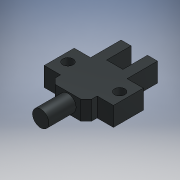
# Autodesk Inventor part: RX670-NW
Saved by Autodesk Inventor 2017 (Build 210142000, 142)
## iProperties
Part Number: RX670-NW
Material: SS41
Document SubType Name: Modeling
Designer: G
Density: 7.85 g/cm^3
Appearance: 鐵灰色
Author: G
Autodesk Inventor part; units mm, degrees
ref_plane "YZ Plane" through (0, 0, 0) normal (1, 0, 0) x (0, 1, 0)
ref_plane "XZ Plane" through (0, 0, 0) normal (0, 1, 0) x (-1, 0, 0)
ref_plane "XY Plane" through (0, 0, 0) normal (0, 0, 1) x (1, 0, 0)
sketch "草圖1" plane through (0, 0, 0) normal (0, 0, 1) x (1, 0, 0)
  line L0 (-6.7, 16.7) -> (-3, 16.7)
  line L1 (-3, 16.7) -> (-3, 7.7)
  line L2 (-3, 7.7) -> (3, 7.7)
  line L3 (3, 7.7) -> (3, 16.7)
  line L4 (3, 16.7) -> (6.7, 16.7)
  line L5 (6.7, 16.7) -> (6.7, 5.5)
  line L6 (-6.7, 5.5) -> (-6.7, 16.7)
  line L7 (12.7, -5.5) -> (12.7, 5.5)
  line L8 (-12.7, 5.5) -> (-12.7, -5.5)
  line L9 (12.7, 5.5) -> (6.7, 5.5)
  line L10 (-6.7, 5.5) -> (-12.7, 5.5)
  line L11 (-6.7, -5.5) -> (-6.7, -7.5)
  line L12 (-6.7, -7.5) -> (-4.7, -9.5)
  line L13 (-4.7, -9.5) -> (-1.5, -9.5)
  line L14 (6.7, -5.5) -> (6.7, -7.5)
  line L15 (6.7, -7.5) -> (4.7, -9.5)
  line L16 (4.7, -9.5) -> (1.5, -9.5)
  line L17 (-12.7, -5.5) -> (-6.7, -5.5)
  line L18 (6.7, -5.5) -> (12.7, -5.5)
  circle A0 centre (-9.5, 0) radius 1.9
  circle A1 centre (9.5, 0) radius 1.9
  line L19 (-9.5, 0) -> (9.5, 0) construction
  line L20 (-1.5, -9.5) -> (1.5, -9.5)
  point P0 (0, 0)
  point P1 (0, 7.7)
  point P2 (0, 0)
  point P3 (0, -9.5)
  dimension "d0" = 6
  dimension "d1" = 13.4
  dimension "d2" = 19
  dimension "d3" = 3.8
  dimension "d4" = 11
  dimension "d5" = 9
  dimension "d7" = 11.2
  dimension "d8" = 25.4
  dimension "d9" = 5.5
  dimension "d10" = 26.2
  dimension "d11" = 135
  dimension "d13" = 2
  constraints: 42 end point, 7 perpendicular, 5 collinear, 5 horizontal, 5 parallel, 4 equal length, 3 midpoint, 2 centre point, 2 horizontal alignment, 2 point on line, 2 vertical, 2 vertical alignment, 1 coincident, 1 equal radius
  measures "d0" distance of L1.end L2.end
  measures "d1" distance between parallel lines of L5 L6
  measures "d2" distance of L19.end L19.start
  measures "d3" diameter of A0
  measures "d4" distance of L8.start L8.end
  measures "d5" distance of L0.end L1.end
  measures "d7" distance between parallel lines of L0 L10
  measures "d8" distance between parallel lines of L7 L8
  measures "d9" distance from line of L17 L19.start
  measures "d10" distance between parallel lines of L0 L13
  measures "d11" angle of L13 L12
  measures "d13" horizontal distance of L12.end L11.end
extrude "擠出1" add sketch "草圖1" along normal mid plane 7
sketch "草圖2" plane through (0, 0, 0) normal (0, 0, 1) x (1, 0, 0)
  line L0 (0, -9.5) -> (3, -9.5)
  line L1 (3, -9.5) -> (3, -19.5)
  line L2 (3, -19.5) -> (0, -19.5)
  line L3 (0, -19.5) -> (0, -9.5)
  line L4 (-4.7, -9.5) -> (4.7, -9.5) construction
  point P0 (0, 0)
  dimension "d17" = 3
  dimension "d18" = 10
  constraints: 8 end point, 2 parallel, 1 horizontal, 1 midpoint, 1 perpendicular
  measures "d17" distance of L1.end L2.end
  measures "d18" distance of L0.end L1.end
revolve "迴轉1" add sketch "草圖2" angle 360 about axis through (0, -19.5, 0) along (0, 1, 0)
